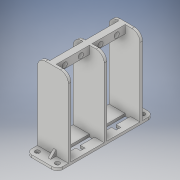
# Autodesk Inventor part: Stewart-Base
Saved by Autodesk Inventor 2018.2 (Build 222227000, 227)
## iProperties
Created: 2018-02-17
Part Number: Stewart-Base
Material: Generisch
Document SubType Name: Modeling
Designer: JochenAlt
Density: 1 g/cm^3
Appearance: Vorgabe
Author: JochenAlt
Autodesk Inventor part; units mm, degrees
ref_plane "YZ Plane" through (0, 0, 0) normal (1, 0, 0) x (0, 1, 0)
ref_plane "XZ Plane" through (0, 0, 0) normal (0, 1, 0) x (-1, 0, 0)
ref_plane "XY Plane" through (0, 0, 0) normal (0, 0, 1) x (1, 0, 0)
sketch "Skizze1" plane through (0, 0, 0) normal (0, 0, 1) x (1, 0, 0)
  line L0 (0, 42.7058) -> (0, -42.7058) construction
  line L1 (-50.7, 0) -> (8.45, 0) construction
  line L2 (-42.25, 21) -> (-10, 21) construction
  line L3 (-10, 21) -> (-10, -21) construction
  line L4 (-10, -21) -> (-42.25, -21) construction
  line L5 (-42.25, -21) -> (-42.25, 21) construction
  line L6 (-16.3, 21) -> (-16.3, -21) construction
  line L7 (-18.8, 21) -> (-18.8, -21) construction
  line L8 (-10, 1.2) -> (-42.25, 1.2) construction
  line L9 (-10, -1.2) -> (-42.25, -1.2) construction
  line L10 (-13.384, 12.1) -> (-16.3, 12.1) construction
  line L11 (-13.384, 10.1) -> (-16.3, 10.1) construction
  line L12 (-10, -10.1) -> (-28.8188, -10.1) construction
  line L13 (-13.384, -12.1) -> (-16.3, -12.1) construction
  line L14 (-13.384, 12.1) -> (-13.384, -12.1) construction
  line L15 (-29.2, 23) -> (-29.2, -23)
  line L16 (-29.2, 21.4) -> (-10, 21.4)
  line L17 (-29.2, 23) -> (-10, 23)
  line L18 (-29.2, -21.4) -> (-10, -21.4)
  line L19 (-29.2, -23) -> (-10, -23)
  line L20 (-10, 23) -> (-10, -23)
  line L21 (-19.2, 21.4) -> (-19.2, -21.4)
  line L22 (-15.9, 21.4) -> (-15.9, -21.4)
  line L23 (-15.9, 12.5) -> (-12.984, 12.5)
  line L24 (-12.984, 12.5) -> (-12.984, 9.7)
  line L25 (-12.984, 9.7) -> (-15.9, 9.7)
  line L26 (-15.9, -9.7) -> (-12.984, -9.7)
  line L27 (-12.984, -9.7) -> (-12.984, -12.5)
  line L28 (-12.984, -12.5) -> (-15.9, -12.5)
  line L29 (-23.2, 21.4) -> (-23.2, -21.4)
  line L30 (-23.2, 21.4) -> (-23.2, 23)
  line L31 (-23.2, -21.4) -> (-23.2, -23)
  line L32 (-19.2, -21.4) -> (-19.2, -23)
  line L33 (-19.2, 21.4) -> (-19.2, 23)
  line L34 (-29.2, 0.8) -> (-10, 0.8)
  line L35 (-29.2, -0.8) -> (-10, -0.8)
  line L36 (-25.8, -29.8) -> (-13.4, -29.8)
  line L37 (-25.8, 29.8) -> (-13.4, 29.8)
  line L38 (-29.2, -23) -> (-29.2, -26.4)
  line L39 (-10, -23) -> (-10, -26.4)
  line L40 (-29.2, 23) -> (-29.2, 26.4)
  line L41 (-10, 23) -> (-10, 26.4)
  arc A0 (-29.2, -26.4) -> (-25.8, -29.8) centre (-25.8, -26.4) ccw
  arc A1 (-13.4, -29.8) -> (-10, -26.4) centre (-13.4, -26.4) ccw
  arc A2 (-10, 26.4) -> (-13.4, 29.8) centre (-13.4, 26.4) ccw
  arc A3 (-25.8, 29.8) -> (-29.2, 26.4) centre (-25.8, 26.4) ccw
  circle A4 centre (-25.8, -26.4) radius 1.4
  circle A5 centre (-13.4, -26.4) radius 1.4
  circle A6 centre (-25.8, 26.4) radius 1.4
  circle A7 centre (-13.4, 26.4) radius 1.4
  point P0 (0, 0)
  point P1 (-15.9, -16.1)
  point P2 (-15.9, -6.1)
  point P3 (-15.9, 6.1)
  point P4 (-15.9, 16.1)
  dimension "d2" = 6.3
  dimension "d3" = 2.5
  dimension "d5" = 2.4
  dimension "d6" = 8.9
  dimension "d7" = 2
  dimension "d9" = 3.384
  dimension "d10" = 32.25
  dimension "d12" = 1.6
  dimension "d13" = 0.4
  dimension "d14" = 0.4
  dimension "d15" = 0.4
  dimension "d16" = 0.4
  dimension "d17" = 0.4
  dimension "d18" = 0.4
  dimension "d27" = 4
  dimension "d30" = 4.9
  dimension "d31" = 10
  dimension "d40" = 19.8
  dimension "d41" = 10
  dimension "d43" = 3.4
  dimension "d45" = 1.6
  dimension "d46" = 10
  dimension "d47" = 2.8
  dimension "d48" = 2
  constraints: 80 end point, 40 point on line, 11 parallel, 10 perpendicular, 8 centre point, 8 horizontal, 8 point on circle, 8 tangent, 8 vertical, 6 equal radius, 4 coincident, 2 symmetric about line, 1 collinear, 10 other
  measures "d2" distance between parallel lines of L3 L6
  measures "d3" distance between parallel lines of L7 L6
  measures "d5" distance between parallel lines of L9 L8
  measures "d6" distance between parallel lines of L10 L2
  measures "d7" distance between parallel lines of L11 L10
  measures "d9" distance between parallel lines of L3 L14
  measures "d10" distance between parallel lines of L5 L3
  measures "d12" distance between parallel lines of L16 L17
  measures "d13" distance between parallel lines of L2 L16
  measures "d14" distance between parallel lines of L7 L21
  measures "d15" distance between parallel lines of L22 L6
  measures "d16" distance between parallel lines of L23 L10
  measures "d17" distance between parallel lines of L11 L25
  measures "d18" distance between parallel lines of L14 L24
  measures "d27" distance between parallel lines of L29 L21
  measures "d30" distance from line of L2 point (-15.9, 16.1)
  measures "d31" distance of point (-15.9, 6.1) point (-15.9, 16.1)
  measures "d40" distance between parallel lines of L8 L2
  measures "d41" distance between parallel lines of L15 L21
  measures "d43" radius of A0
  measures "d45" distance between parallel lines of L34 L35
  measures "d46" distance between parallel lines of L0 L3
  measures "d47" diameter of A4
  measures "d48" distance edge to line of A4 L19
extrude "Extrusion1" add sketch "Skizze1" along normal blind 1.6 contours L17 L30 L16 L15 | L40 A3 L37 A2 L41 L17 | L16 L29 L34 L15 | L17 L33 L16 L30 | L34 L29 L35 L15 | L16 L21 L34 L29 | L17 L20 L16 L33 | L35 L29 L18 L15 | L34 L21 L35 L29 | L18 L31 L19 L15 | L35 L21 L18 L29 | L16 L20 L34 L22 L25 L24 L23 | L19 L39 A1 L36 A0 L38 | L18 L32 L19 L31 | L34 L20 L35 L22 | L18 L20 L19 L32 | L35 L20 L18 L22 L28 L27 L26
extrude "Extrusion2" add sketch "Skizze1" along normal blind 42.7 contours L17 L30 L16 L15 | L17 L33 L16 L30 | L34 L29 L35 L15 | L17 L20 L16 L33 | L34 L21 L35 L29 | L18 L31 L19 L15 | L34 L22 L35 L21 | L18 L32 L19 L31 | L34 L20 L35 L22 | L18 L20 L19 L32
extrude "Extrusion4" add sketch "Skizze1" along normal blind 1.6 from surface at 42.7 contours L17 L30 L16 L15 | L17 L33 L16 L30 | L34 L29 L35 L15 | L17 L20 L16 L33 | L34 L21 L35 L29 | L18 L31 L19 L15 | L34 L22 L35 L21 | L18 L32 L19 L31 | L34 L20 L35 L22 | L18 L20 L19 L32
extrude "Extrusion5" add sketch "Skizze1" along normal blind 5 from surface at 44.3 contours L17 L30 L16 L15 | L17 L33 L16 L30 | L34 L29 L35 L15 | L16 L21 L34 L29 | L17 L20 L16 L33 | L34 L21 L35 L29 | L18 L31 L19 L15 | L35 L21 L18 L29 | L34 L22 L35 L21 | L18 L32 L19 L31 | L34 L20 L35 L22 | L18 L20 L19 L32
sketch "Skizze2" plane through (-23.2, -23, 49.3) normal (-1, 0, 0) x (0, 0, 1)
  line L0 (-49.3, 16.9) -> (0, 16.9) construction
  line L1 (0, 23.8) -> (0, 44.4) projected
  line L2 (-49.3, 6.9) -> (0, 6.9) construction
  line L3 (-60.36, 23) -> (10.06, 23) construction
  line L4 (-49.3, 64.72) -> (-49.3, -18.72) construction
  line L5 (-49.3, 29.1) -> (0, 29.1) construction
  line L6 (-49.3, 39.1) -> (0, 39.1) construction
  circle A0 centre (-3, 39.1) radius 1.6
  circle A1 centre (-3, 29.1) radius 1.6
  circle A2 centre (-3, 16.9) radius 1.6
  circle A3 centre (-3, 6.9) radius 1.6
  line L7 (-3, 39.1) -> (-3, 6.9) construction
  line L8 (-49.3, 49.4) -> (-49.3, -3.4) construction
  line L9 (-5, 23.8) -> (-5, 44.4) construction
  line L10 (-6.6, 44.4) -> (-6.6, 1.6) construction
  point P0 (-49.3, 23)
  point P1 (0, 0)
  point P2 (0, 46)
  point P3 (-49.3, 46)
  point P4 (-49.3, 0)
  point P5 (-5, 0)
  point P6 (-5, 46)
  point P7 (-50.3, 44.4)
  point P8 (-50.3, 1.6)
  point P9 (-6, 44.4)
  point P10 (-7.6, 22.2084)
  point P11 (-7.6, 23.866)
  point P12 (-5, 22.2084)
  point P13 (-5, 1.6)
  dimension "d32" = 3.2
  dimension "d34" = 3.6
  constraints: 10 end point, 10 point on line, 4 centre point, 3 equal radius, 3 horizontal, 1 parallel, 1 vertical, 4 other
  measures "d32" diameter of A0
extrude "Extrusion6" cut sketch "Skizze2" against normal blind 20
fillet "Rundung2" radius 5 6 edges at (-29.2, 0, 49.3) (-29.2, 22.2, 49.3) (-10, 22.2, 49.3) (-10, 0, 49.3) (-29.2, -22.2, 49.3) (-10, -22.2, 49.3)
sketch "Skizze3" plane through (-19.2, 0, 0) normal (1, 0, 0) x (0, 1, 0)
  line L0 (-23, 1.6) -> (-26.4, 1.6) projected
  line L1 (-26.4, 1.6) -> (-23, 5)
  line L2 (-23, 1.6) -> (-23, 5)
  line L3 (-23, 1.6) -> (-26.4, 1.6)
  line L4 (26.4, 1.6) -> (23, 5)
  line L5 (23, 1.6) -> (23, 44.3) construction
  line L6 (-23, 5) -> (23, 5) construction
  line L7 (0, 59.16) -> (0, -9.86) construction
  line L8 (-41.72, 0) -> (41.72, 0) construction
  line L9 (23, 5) -> (23, 1.6)
  line L10 (23, 1.6) -> (26.4, 1.6)
  point P0 (0, 0)
  dimension "d49" = 45
  constraints: 14 end point, 2 collinear, 1 horizontal, 1 parallel, 1 point on line, 1 vertical
  measures "d49" angle of L0 L1
extrude "Extrusion8" add sketch "Skizze3" along normal blind 1.6
equation "\"d5\" = d11 + 2 * d13"
equation "\"d12\" = d11"
equation "\"d14\" = d13"
equation "\"d15\" = d13"
equation "\"d16\" = d13"
equation "\"d17\" = d13"
equation "\"d18\" = d13"
equation "\"d25\" = d11"
equation "\"d11\" = 1.6"
